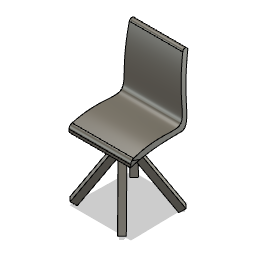
Chair (Autodesk Fusion 360 design; units mm, degrees)
Autodesk Fusion 360 part; units mm, degrees
sketch "Sketch3" plane through (0, 0, 0) normal (1, 0, 0) x (0, 0, -1)
  line L0 (0, 0) -> (30, 0) construction
  line L1 (30, 0) -> (30, 35) construction
  line L2 (30, 35) -> (0, 35) construction
  line L3 (0, 35) -> (0, 0) construction
  spline S0 degree 5 poles (0, 0) (-0.0769, 0.0223) (-0.117, 0.0898) (0.1648, 0.2601) (1.2221, 0.6212) (3.6163, 1.2581) (6.7684, 1.8644) (10.3209, 2.3143) (13.9509, 2.5834) (17.3689, 2.7059) (20.3544, 2.7258) (22.7703, 2.7243) (24.6036, 2.6425) (25.9575, 2.6851) (26.9633, 3.3706) (27.6552, 4.894) (27.9992, 7.0923) (28.0895, 9.9629) (28.0531, 13.4893) (28.0556, 17.6998) (28.2649, 22.6285) (28.7197, 27.1792) (29.2723, 30.949) (29.7408, 33.6229) (30, 35) knots 0 0 0 0 0 0 0.05 0.1 0.15 0.2 0.25 0.3 0.35 0.4 0.45 0.5 0.55 0.6 0.65 0.7 0.75 0.8 0.85 0.9 0.95 1 1 1 1 1 1
  spline S1 degree 5 poles (0, 2.9958) (-0.1843, 2.9296) (-0.3968, 2.8498) (-0.2482, 2.8875) (0.8973, 3.2615) (3.6285, 4.0716) (6.9387, 4.7603) (10.4142, 5.1877) (13.7303, 5.3211) (16.7043, 5.2513) (19.2437, 5.1087) (21.3318, 5.0405) (23.0244, 5.1188) (24.3278, 5.463) (25.23, 6.2213) (25.7408, 7.5273) (25.9286, 9.4682) (25.9047, 12.0927) (25.8071, 15.4216) (25.7844, 19.4557) (25.9808, 24.184) (26.4125, 28.5093) (26.9303, 32.0521) (27.3664, 34.5459) (27.6072, 35.8258) knots 0 0 0 0 0 0 0.05 0.1 0.15 0.2 0.25 0.3 0.35 0.4 0.45 0.5 0.55 0.6 0.65 0.7 0.75 0.8 0.85 0.9 0.95 1 1 1 1 1 1
  line L4 (27.6072, 35.8258) -> (30, 35)
  line L5 (0, 2.9958) -> (0, 0)
  line L6 (-9.8215, 2.9958) -> (54.9422, 2.9958) construction
  line L7 (-4.9886, 1.5537) -> (8.5806, 5.4763)
  line L8 (-3.8186, -0.5735) -> (9.9153, 2.7266)
  line L9 (14.7801, 5.1743) -> (26.4044, 4.9877)
  line L10 (16.7482, 2.8007) -> (28.3725, 2.6142)
  line L11 (25.3432, 23.7917) -> (29.8711, 47.8599)
  line L12 (27.7346, 22.9662) -> (32.2654, 47.0338)
  line L13 (25.3535, 1.3206) -> (28.6016, 6.0917)
  point P0 (3.0483, 1.0766)
  point P1 (22.5604, 2.7075)
  point P2 (26.9775, 3.7062)
  point P3 (1.796, 3.515)
  point P4 (20.5922, 5.081)
  point P5 (25.145, 6.3761)
  dimension "d10" = 30
  dimension "d11" = 35
  constraint horizontal L0
  constraint vertical L1
  constraint horizontal L2
  constraint vertical L3
  constraint coincident L0.start L3.end
  constraint horizontal L6
  constraint midpoint P3 L7
  constraint midpoint P0 L8
  constraint equal L7 L8
  constraint midpoint P4 L9
  constraint midpoint P1 L10
  constraint equal L9 L10
  constraint midpoint S1.end L11
  constraint midpoint L1.end L12
  constraint equal L11 L12
  constraint coincident S1.start L7
  constraint coincident S1.start L6
  constraint midpoint P2 L13
  measures "d10" distance of L0.start L0.end
  measures "d11" distance of L0.start L2.end
extrude "Extrude4" add sketch "Sketch3" along normal blind 30 contours S0 L5 L8 | S0 S1 L4 L5 L8 L10 | S0 L10 makes body 1
fillet "Fillet1" radius 2 1 edges at (15, 2.9707, 0) on bodies 1
move_body "Move1" bodies 1 to x (1, 0, 0) y (0, 1, 0) z (0, 0, 1) at (0, -2.5, 0)
chamfer "Chamfer1" distance 40 angle 3 1 edges at (0, 32.9129, -28.8036) measured on face at (0, 0.188, -6.7602) on bodies 1
chamfer "Chamfer2" distance 40 angle 3 1 edges at (30, 32.9129, -28.8036) measured on face at (30, 0.188, -6.7602) on bodies 1
fillet "Fillet2" radius 1.3 2 edges at (15, 33.3258, -27.6072) (15, 32.5, -30) on bodies 1
sketch "Sketch5" plane through (0, 0, 0) normal (1, 0, 0) x (0, 0, -1)
ref_plane "WorkPlane1" through (15, 15.4767, -15) normal (1, 0, 0) x (0, 0, -1)
ref_plane "WorkPlane2" through (0, 0, -30) normal (0, 0, 1) x (1, 0, 0)
ref_plane "WorkPlane3" through (0, 0, -15) normal (0, 0, 1) x (1, 0, 0)
ref_plane "WorkPlane4" through (0, 2, 0) normal (0, 1, 0) x (0, 0, 1)
ref_plane "WorkPlane5" through (0, -26, 0) normal (0, 1, 0) x (0, 0, 1)
ref_plane "WorkPlane6" through (4.3934, 0, -25.6066) normal (-0.707107, 0, 0.707107) x (0.707107, 0, 0.707107)
ref_plane "WorkPlane7" through (3.3327, 0, -24.5459) normal (-0.707107, 0, 0.707107) x (0.707107, 0, 0.707107)
sketch "Sketch6" plane through (3.3327, 0, -24.5459) normal (-0.707107, 0, 0.707107) x (0.707107, 0, 0.707107)
  line L0 (13.1544, 1.7423, -0.2417) -> (35.8558, -31.3964, 0)
  line L1 (35.8558, -31.3964, 0) -> (35.8836, -31.3555, 2.9996)
  line L2 (35.8836, -31.3555, 2.9996) -> (13.1821, 1.7832, 2.7579)
  line L3 (13.1821, 1.7832, 2.7579) -> (13.1544, 1.7423, -0.2417)
  dimension "d19" = 3
extrude "Extrude5" add sketch "Sketch6" against normal blind 3 separate body contours L0 L1 L2 L3 in plane through (10.3675, 6.6895, -17.768) normal (0.594168, 0.565009, 0.572476) makes body 2
sketch "Sketch7" plane through (15, 18.7685, -13.6803) normal (1, 0, 0) x (0, 0, -1)
  line L0 (0, -37.4353) -> (0, -3.8537) construction
  constraint vertical L0
pattern_circular "C-Pattern1" count 4 over 360 about axis through (15, -18.6668, -13.6803) along (0, 1, 0) of bodies 2 makes body 3 at (18.1003, -9.869, -16.1851) makes body 4 at (12.4952, -9.869, -16.7806) makes body 5 at (4.4924, -20.3229, -6.6884)
combine "Combine1" operation cut target body 2 tool bodies 3 4 5 keep tools
combine "Combine2" operation cut target body 3 tool bodies 2 4 5 keep tools
combine "Combine3" operation cut target body 4 tool bodies 2 3 5 keep tools
combine "Combine4" operation cut target body 5 tool bodies 2 3 4 keep tools
combine "Combine5" operation cut target body 2 tool bodies 1 keep tools
combine "Combine6" operation cut target body 3 tool bodies 1 keep tools
combine "Combine7" operation cut target body 4 tool bodies 1 keep tools
combine "Combine8" operation cut target body 5 tool bodies 1 keep tools
sketch "Sketch8" plane through (0, 0, 0) normal (0, 0, 1) x (1, 0, 0)
  line L0 (-3.219, 33.7971) -> (34.781, 33.7971) construction
  line L1 (34.781, 33.7971) -> (34.781, -34.2029) construction
  line L2 (34.781, -34.2029) -> (-3.219, -34.2029) construction
  line L3 (-3.219, -34.2029) -> (-3.219, 33.7971) construction
  line L4 (-3.219, -34.2029) -> (34.781, -34.2029) construction
  line L5 (34.781, -34.2029) -> (34.781, 0.7971) construction
  line L6 (34.781, 0.7971) -> (-3.219, 0.7971) construction
  line L7 (-3.219, 0.7971) -> (-3.219, -34.2029) construction
  dimension "d29" = 38
  dimension "d30" = 68
  dimension "d31" = 38
  dimension "d32" = 35
  constraint horizontal L0
  constraint vertical L1
  constraint horizontal L2
  constraint vertical L3
  constraint horizontal L4
  constraint vertical L5
  constraint horizontal L6
  constraint vertical L7
  measures "d29" distance of L0.start L0.end
  measures "d30" distance of L0.start L2.end
  measures "d31" distance of L2.end L1.end
  measures "d32" distance of L2.end L6.end
sketch "Sketch9" plane through (0, 0, 0) normal (1, 0, 0) x (0, 0, -1)
  line L0 (27.6053, 33.3766) -> (0, 0)
  line L1 (27.6053, 33.3766) -> (0, 0)
  line L2 (0, 0, 0) -> (0, 0, 29.7676)
  line L3 (0, 0, 29.7676) -> (27.6053, 33.3766, 29.7676)
  line L4 (27.6053, 33.3766, 29.7676) -> (27.6053, 33.3766, 0)
  constraint coincident L0.end L1.end
sketch "Sketch11" plane through (14.8838, 16.6883, -13.8026) normal (0, 0.637338, 0.770584) x (1, 0, 0)
  line L0 (-11.5052, 26.3273) -> (-8.5052, 26.3273)
  line L1 (-8.5052, 26.3273) -> (-8.5052, 21.3273)
  line L2 (-8.5052, 21.3273) -> (-11.5052, 21.3273)
  line L3 (-11.5052, 21.3273) -> (-11.5052, 26.3273)
  line L4 (11.0029, 26.4672) -> (8.0029, 26.4672)
  line L5 (8.0029, 26.4672) -> (8.0029, 21.4672)
  line L6 (8.0029, 21.4672) -> (11.0029, 21.4672)
  line L7 (11.0029, 21.4672) -> (11.0029, 26.4672)
  line L8 (-13.7405, -28.2921) -> (-10.7405, -28.2921)
  line L9 (-10.7405, -28.2921) -> (-10.7405, -22.2921)
  line L10 (-10.7405, -22.2921) -> (-13.7405, -22.2921)
  line L11 (-13.7405, -22.2921) -> (-13.7405, -28.2921)
  line L12 (9.9429, -28.3461) -> (12.9429, -28.3461)
  line L13 (12.9429, -28.3461) -> (12.9429, -22.3461)
  line L14 (12.9429, -22.3461) -> (9.9429, -22.3461)
  line L15 (9.9429, -22.3461) -> (9.9429, -28.3461)
  dimension "d39" = 3
  dimension "d40" = 5
  dimension "d41" = 3
  dimension "d42" = 5
  dimension "d43" = 3
  dimension "d44" = 6
  dimension "d45" = 3
  dimension "d46" = 6
  constraint horizontal L0
  constraint vertical L1
  constraint horizontal L2
  constraint vertical L3
  constraint horizontal L4
  constraint vertical L5
  constraint horizontal L6
  constraint vertical L7
  constraint horizontal L8
  constraint vertical L9
  constraint horizontal L10
  constraint vertical L11
  constraint horizontal L12
  constraint vertical L13
  constraint horizontal L14
  constraint vertical L15
  measures "d39" distance of L0.start L0.end
  measures "d40" distance of L0.start L2.end
  measures "d41" distance of L4.start L4.end
  measures "d42" distance of L4.start L6.end
  measures "d43" distance of L8.start L8.end
  measures "d44" distance of L8.start L10.end
  measures "d45" distance of L12.start L12.end
  measures "d46" distance of L12.start L14.end
extrude "Extrude7" add sketch "Sketch11" against normal blind 3 separate body makes body 6 at (25.8867, 34.5246, -31.1502) makes body 7 at (1.1433, -4.8466, 1.4131) makes body 8 at (3.3786, 33.7697, -29.2281) makes body 9 at (24.8267, -4.8882, 1.4475)
sketch "Sketch10" plane through (14.8838, 16.6883, -13.8026) normal (0, 0.637338, 0.770584) x (1, 0, 0)
  line L0 (-18.8074, 26.124) -> (19.1926, 26.124)
  line L1 (19.1926, 26.124) -> (19.1926, -27.876)
  line L2 (19.1926, -27.876) -> (-18.8074, -27.876)
  line L3 (-18.8074, -27.876) -> (-18.8074, 26.124)
  dimension "d33" = 38
  dimension "d34" = 54
  constraint horizontal L0
  constraint vertical L1
  constraint horizontal L2
  constraint vertical L3
  measures "d33" distance of L0.start L0.end
  measures "d34" distance of L0.start L2.end
extrude "Extrude6" add sketch "Sketch10" against normal blind 20 separate body makes body 10
hidden bodies 6 7 8 9 10
named bodies: "Stoelleuning", "Poot1", "Poot2", "Poot3", "Poot4", "Stock", "Helper1", "Helper2", "Helper3", "Helper4"
